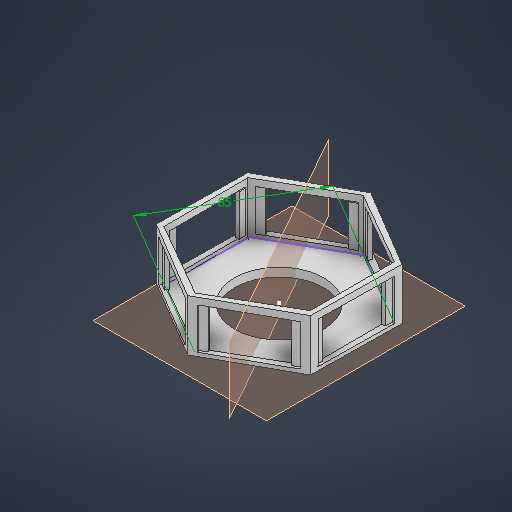
# Autodesk Inventor part: Part1
Saved by Autodesk Inventor 2027 (Build 310192060, 192F)
## iProperties
Created: 2026-07-17
Part Number: Part1
Material: Generic
Document SubType Name: Modeling
Designer: farde
Density: 1 g/cm^3
Appearance: Default
Author: farde
Autodesk Inventor part; units mm, degrees
ref_plane "YZ Plane" through (0, 0, 0) normal (1, 0, 0) x (0, 1, 0)
ref_plane "XY Plane" through (0, 0, 0) normal (0, 0, 1) x (1, 0, 0)
sketch "Sketch1" plane through (0, 0, 0) normal (0, 1, 0) x (-1, 0, 0)
  line L0 (-42.7114, -24.1674) -> (-42.2853, 24.9055)
  line L1 (-42.2853, 24.9055) -> (0.4261, 49.0729)
  line L2 (0.4261, 49.0729) -> (42.7114, 24.1674)
  line L3 (42.7114, 24.1674) -> (42.2853, -24.9055)
  line L4 (42.2853, -24.9055) -> (-0.4261, -49.0729)
  line L5 (-0.4261, -49.0729) -> (-42.7114, -24.1674)
  point P0 (0, 0)
  point P1 (0, 0)
  dimension "d0" = 85
  constraints: 12 end point, 1 coincident, 13 other
  measures "d0" distance between parallel lines of L5 L2
sketch "Sketch2" plane through (0, 0, 0) normal (0, 1, 0) x (-1, 0, 0)
  line L0 (-46.0208, -25.7239) -> (-45.288, 26.9933)
  line L1 (-45.288, 26.9933) -> (0.7329, 52.7172)
  line L2 (0.7329, 52.7172) -> (46.0208, 25.7239)
  line L3 (46.0208, 25.7239) -> (45.288, -26.9933)
  line L4 (45.288, -26.9933) -> (-0.7329, -52.7172)
  line L5 (-0.7329, -52.7172) -> (-46.0208, -25.7239)
  point P0 (0, 0)
  point P1 (0, 0)
  dimension "d1" = 52.7172
  constraints: 12 end point, 1 coincident, 13 other
  measures "d1" vertical distance of L2.end L3.end
extrude "Extrusion1" add sketch "Sketch2" along normal blind 30
sketch "Sketch3" plane through (0, 0, 0) normal (0, -1, 0) x (1, 0, 0)
  line L0 (42.7068, 24.4765) -> (42.5507, -24.7469)
  line L1 (42.5507, -24.7469) -> (-0.1561, -49.2235)
  line L2 (-0.1561, -49.2235) -> (-42.7068, -24.4765)
  line L3 (-42.7068, -24.4765) -> (-42.5507, 24.7469)
  line L4 (-42.5507, 24.7469) -> (0.1561, 49.2235)
  line L5 (0.1561, 49.2235) -> (42.7068, 24.4765)
  point P0 (0, 0)
  point P1 (0, 0)
  constraints: 12 end point, 1 coincident, 13 other
extrude "Extrusion2" cut sketch "Sketch3" against normal blind 49.1375
ref_plane "Work Plane1" through (0, -5, 0) normal (0, 1, 0) x (-1, 0, 0)
sketch "Sketch4" plane through (0, -5, 0) normal (0, 1, 0) x (-1, 0, 0)
  circle A0 centre (0, 0) radius 26
  dimension "d7" = 52
  constraints: 1 centre point, 1 coincident
  measures "d7" diameter of A0
loft "Loft1" add profiles "Sketch4" section 2 edges at (-42.6288, 0, 0.1352) (-21.1973, 0, 36.9852) (21.4315, 0, 36.85) (42.6288, 0, -0.1352) (21.1973, 0, -36.9852) (-21.4315, 0, -36.85)
sketch "Sketch5" plane through (0, -5, 0) normal (0, -1, 0) x (0.999995, 0, -0.0031715)
  circle A0 centre (0, 0) radius 26
  constraints: 1 centre point, 1 coincident
extrude "Extrusion3" cut sketch "Sketch5" against normal blind 73.1
sketch "Sketch6" plane through (-45.288, 0, -26.9933) normal (-0.4879136, 0, -0.8728919) x (-0.8728919, 0, 0.4879136)
  line L0 (-48.3611, 26.134) -> (-4.3611, 26.134)
  line L1 (-4.3611, 26.134) -> (-4.3611, 2.134)
  line L2 (-4.3611, 2.134) -> (-48.3611, 2.134)
  line L3 (-48.3611, 2.134) -> (-48.3611, 26.134)
  line L4 (-48.3611, 26.134) -> (-4.3611, 2.134) construction
  line L5 (-4.3611, 26.134) -> (-48.3611, 2.134) construction
  point P0 (-26.3611, 0)
  point P1 (-26.3611, 14.134)
  dimension "d14" = 44
  dimension "d15" = 24
  constraints: 12 end point, 2 midpoint, 2 parallel, 1 horizontal, 1 perpendicular
  measures "d14" distance of L1.end L2.end
  measures "d15" distance of L0.end L1.end
extrude "Extrusion4" cut sketch "Sketch6" against normal blind 26.9125
pattern_circular "Circular Pattern1" count 6 over 360 about axis through (0, -5, 0) along (0, 1, 0) of "Extrusion4"
sketch "Sketch7" plane through (-41.4812, 2.134, -29.1211) normal (0.8728919, 0, -0.4879136) x (-0.4879136, 0, -0.8728919)
  line L0 (-3.3993, 0) -> (-3.3993, 24) projected
  line L1 (0, 0) -> (-3.3993, 0) projected
  line L2 (-3.3993, 24) -> (-1.3993, 24)
  line L3 (-1.3993, 24) -> (-1.3993, 0)
  line L4 (-1.3993, 0) -> (-3.3993, 0)
  line L5 (-3.3993, 0) -> (-3.3993, 24)
  point P0 (-45.6588, -2.134)
  dimension "d21" = 2
  constraints: 8 end point, 2 parallel, 1 horizontal, 1 perpendicular, 1 point on line
  measures "d21" distance of L3.end L4.end
extrude "Extrusion5" add sketch "Sketch7" along normal blind 4
ref_plane "Work Plane2" through (-22.2776, 2.134, -39.8552) normal (0.8728919, 0, -0.4879136) x (-0.4879136, 0, -0.8728919)
mirror "Mirror1" about plane through (-22.2776, 2.134, -39.8552) normal (0.8728919, 0, -0.4879136) of "Extrusion5"
pattern_circular "Circular Pattern2" count 6 over 360 about axis through (0, -10, 0) along (0, 1, 0) of "Extrusion5"
pattern_circular "Circular Pattern3" count 6 over 360 about axis through (0, -10, 0) along (0, 1, 0) of "Extrusion5", "Mirror1"
body "Solid1"
